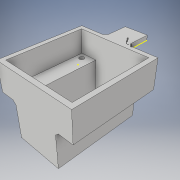
# Autodesk Inventor part: obudowa_baza
Saved by Autodesk Inventor 2019 (Build 230136000, 136)
## iProperties
Created: 2019-08-12
Part Number: obudowa_baza
Material: Ogólny
Document SubType Name: Modeling
Designer: mikol
Density: 1 g/cm^3
Appearance: Domyślna
Author: mikol
Autodesk Inventor part; units mm, degrees
ref_plane "YZ Plane" through (0, 0, 0) normal (1, 0, 0) x (0, 1, 0)
ref_plane "XZ Plane" through (0, 0, 0) normal (0, 1, 0) x (-1, 0, 0)
ref_plane "XY Plane" through (0, 0, 0) normal (0, 0, 1) x (1, 0, 0)
sketch "Sketch1" plane through (0, 0, 0) normal (0, 1, 0) x (-1, 0, 0)
  circle A0 centre (0, 12.75) radius 8.05
  circle A1 centre (0, -12.75) radius 8.05
  line L0 (14.5, 27) -> (-14.5, 27)
  line L1 (-14.5, 27) -> (-14.5, -27)
  line L2 (-14.5, -27) -> (14.5, -27)
  line L3 (14.5, -27) -> (14.5, 27)
  line L4 (14.5, 27) -> (-14.5, -27) construction
  line L5 (-14.5, 27) -> (14.5, -27) construction
  point P0 (0, 0)
  dimension "d0" = 16.1
  dimension "d1" = 16.1
  dimension "d2" = 25.5
  dimension "d3" = 29
  dimension "d4" = 54
  dimension "d5" = 14.5
  dimension "d6" = 14.5
  dimension "d7" = 14.25
  dimension "d8" = 14.25
  constraints: 12 end point, 2 centre point, 2 midpoint, 2 parallel, 1 horizontal, 1 perpendicular
  measures "d0" diameter of A0
  measures "d1" diameter of A1
  measures "d2" distance of A1.centre A0.centre
  measures "d3" distance of L2.end L1.end
  measures "d4" distance of L1.end L0.end
  measures "d5" distance from line of L3 A0.centre
  measures "d6" distance from line of A1.centre L3
  measures "d7" distance from line of L2 A1.centre
  measures "d8" distance from line of L0 A0.centre
extrude "Extrusion1" add sketch "Sketch1" along normal blind 3
sketch "Sketch2" plane through (0, 3, 0) normal (0, 1, 0) x (1, 0, 0)
  line L0 (-11.5, -24) -> (11.5, -24)
  line L1 (11.5, -24) -> (11.5, 24)
  line L2 (11.5, 24) -> (-11.5, 24)
  line L3 (-11.5, 24) -> (-11.5, -24)
  line L4 (-11.5, -24) -> (11.5, 24) construction
  line L5 (11.5, -24) -> (-11.5, 24) construction
  line L6 (14.5, -27) -> (14.5, 27) projected
  line L7 (-14.5, -27) -> (14.5, -27)
  line L8 (14.5, -27) -> (14.5, 27)
  line L9 (14.5, 27) -> (-14.5, 27)
  line L10 (-14.5, 27) -> (-14.5, -27)
  line L11 (-14.5, -27) -> (14.5, 27) construction
  line L12 (14.5, -27) -> (-14.5, 27) construction
  point P0 (0, 0)
  dimension "d11" = 23
  dimension "d12" = 48
  constraints: 24 end point, 4 midpoint, 4 parallel, 2 horizontal, 2 perpendicular
  measures "d11" distance of L2.end L1.end
  measures "d12" distance of L1.end L0.end
extrude "Extrusion2" add sketch "Sketch2" along normal blind 25
sketch "Sketch3" plane through (0, 28, 0) normal (0, 1, 0) x (1, 0, 0)
  line L0 (-25.5, 27) -> (25.5, 27)
  line L1 (25.5, 27) -> (25.5, -27)
  line L2 (25.5, -27) -> (-25.5, -27)
  line L3 (-25.5, -27) -> (-25.5, 27)
  line L4 (-25.5, 27) -> (25.5, -27) construction
  line L5 (25.5, 27) -> (-25.5, -27) construction
  line L6 (14.5, -27) -> (14.5, 27) projected
  line L7 (-14.5, 27) -> (14.5, 27)
  line L8 (14.5, 27) -> (14.5, -27)
  line L9 (14.5, -27) -> (-14.5, -27)
  line L10 (-14.5, -27) -> (-14.5, 27)
  line L11 (-14.5, 27) -> (14.5, -27) construction
  line L12 (14.5, 27) -> (-14.5, -27) construction
  point P0 (0, 0)
  dimension "d15" = 51
  constraints: 24 end point, 4 midpoint, 4 parallel, 2 horizontal, 2 perpendicular
  measures "d15" distance of L1.end L2.end
extrude "Extrusion3" add sketch "Sketch3" against normal blind 3 contours L0 L10 L2 L3 | L0 L1 L2 L6
sketch "Sketch4" plane through (0, 28, 0) normal (0, 1, 0) x (1, 0, 0)
  line L0 (-25.5, -27) -> (25.5, -27) projected
  line L1 (-25.5, 27) -> (25.5, 27)
  line L2 (25.5, 27) -> (25.5, -27)
  line L3 (25.5, -27) -> (-25.5, -27)
  line L4 (-25.5, -27) -> (-25.5, 27)
  line L5 (-25.5, 27) -> (25.5, -27) construction
  line L6 (25.5, 27) -> (-25.5, -27) construction
  line L7 (-22.5, 24) -> (22.5, 24)
  line L8 (22.5, 24) -> (22.5, -24)
  line L9 (22.5, -24) -> (-22.5, -24)
  line L10 (-22.5, -24) -> (-22.5, 24)
  line L11 (-22.5, 24) -> (22.5, -24) construction
  line L12 (22.5, 24) -> (-22.5, -24) construction
  point P0 (0, 0)
  dimension "d18" = 45
  dimension "d19" = 48
  constraints: 24 end point, 4 midpoint, 4 parallel, 2 horizontal, 2 perpendicular
  measures "d18" distance of L8.end L9.end
  measures "d19" distance of L7.end L8.end
extrude "Extrusion4" add sketch "Sketch4" along normal blind 15
sketch "Sketch5" plane through (0, 28, 0) normal (0, 1, 0) x (1, 0, 0)
  line L0 (-11.5, 24) -> (-22.5, 24) projected
  line L1 (-22.5, 24) -> (-22.5, -24) projected
  line L2 (-22.5, -24) -> (-11.5, -24) projected
  line L3 (-11.5, -24) -> (-11.5, 24) projected
  line L4 (22.5, 24) -> (11.5, 24) projected
  line L5 (11.5, 24) -> (11.5, -24) projected
  line L6 (11.5, -24) -> (22.5, -24) projected
  line L7 (22.5, -24) -> (22.5, 24) projected
  circle A0 centre (18.5, 20) radius 1.75
  line L8 (14.5, 27) -> (14.5, -27) projected
  line L9 (14.5, 27) -> (25.5, 27) projected
  line L10 (25.5, 27) -> (25.5, -27) projected
  line L11 (25.5, -27) -> (14.5, -27) projected
  line L12 (-11.5, 24) -> (-11.5, -24) projected
  line L13 (-11.5, -24) -> (11.5, -24) projected
  line L14 (11.5, -24) -> (11.5, 24) projected
  line L15 (11.5, 24) -> (-11.5, 24) projected
  circle A1 centre (0, 12.75) radius 8.05 projected
  circle A2 centre (0, -12.75) radius 8.05 projected
  circle A3 centre (18.5, -20) radius 1.75
  circle A4 centre (-18.5, 20) radius 1.75
  circle A5 centre (-18.5, -20) radius 1.75
  point P0 (0, 0)
  dimension "d22" = 3.5
  dimension "d23" = 4
  dimension "d24" = 4
  dimension "d25" = 4
  dimension "d28" = 40
  dimension "d31" = 37
  dimension "d53" = 4
  constraints: 4 centre point, 1 horizontal, 1 vertical, 6 other
  measures "d22" diameter of A0
  measures "d23" distance from line of L7 A0.centre
  measures "d24" distance from line of L8 A0.centre
  measures "d25" distance from line of L4 A0.centre
  measures "d28" distance of A0.centre A3.centre
  measures "d31" distance of A0.centre A4.centre
  measures "d53" distance from line of L6 A3.centre
extrude "Extrusion5" cut sketch "Sketch5" against normal blind 10 contours A0 | A3 | A4 | A5
chamfer "Chamfer1" distance 2 angle 45 4 edges at (-14.5, 0, 0) (14.5, 0, 0) (0, 0, 27) (0, 0, -27)
chamfer "Chamfer2" distance 2 angle 45 2 edges at (-14.5, 25, 0) (14.5, 25, 0)
sketch "Sketch6" plane through (0, 25, 0) normal (0, -1, 0) x (1, 0, 0)
  line L0 (-16.5, 27) -> (-16.5, -27) projected
  circle A0 centre (-18.5, -20) radius 1.75 projected
  circle A1 centre (-18.5, 20) radius 1.75 projected
  line L1 (-16.5, 27) -> (-25.5, 27) projected
  line L2 (-25.5, 27) -> (-25.5, -27) projected
  line L3 (-25.5, -27) -> (-16.5, -27) projected
  line L4 (16.5, -27) -> (16.5, 27) projected
  circle A2 centre (18.5, -20) radius 1.75 projected
  line L5 (16.5, -27) -> (25.5, -27) projected
  line L6 (25.5, -27) -> (25.5, 27) projected
  line L7 (25.5, 27) -> (16.5, 27) projected
  circle A3 centre (18.5, 20) radius 1.75 projected
  circle A4 centre (18.5, -20) radius 3
  circle A5 centre (18.5, 20) radius 3
  circle A6 centre (-18.5, -20) radius 3
  circle A7 centre (-18.5, 20) radius 3
  point P0 (0, 0)
  dimension "d42" = 6
  dimension "d45" = 40
  dimension "d48" = 37
  constraints: 4 centre point, 1 coincident, 1 horizontal, 1 vertical, 6 other
  measures "d42" diameter of A4
  measures "d45" distance of A4.centre A5.centre
  measures "d48" distance of A4.centre A6.centre
extrude "Extrusion6" cut sketch "Sketch6" along normal blind 10 contours A7 L0 | L0 A7 | A6 L0 | L0 A6 | A0 | A1 | A4 L4 | L4 A4 | A5 L4 | L4 A5 | A2 | A3
sketch "Sketch7" plane through (25.5, 43, -27) normal (0, 0, -1) x (-1, 0, 0)
  line L0 (40, -41) -> (11, -41) projected
  line L1 (40, -41) -> (40, -20) projected
  line L2 (42, -18) -> (40, -20) projected
  line L3 (51, -18) -> (42, -18) projected
  line L4 (51, 0) -> (51, -18) projected
  line L5 (0, 0) -> (51, 0) projected
  line L6 (0, -18) -> (0, 0) projected
  line L7 (9, -18) -> (0, -18) projected
  line L8 (11, -20) -> (9, -18) projected
  line L9 (11, -41) -> (11, -20) projected
  line L10 (0, 0) -> (51, 0) projected
  line L11 (18, 0) -> (33, 0)
  line L12 (33, 0) -> (33, -3)
  line L13 (33, -3) -> (18, -3)
  line L14 (18, -3) -> (18, 0)
  point P0 (25.5, -43)
  dimension "d54" = 15
  dimension "d55" = 3
  dimension "d56" = 18
  dimension "d57" = 18
  constraints: 8 end point, 2 parallel, 1 horizontal, 1 perpendicular, 1 point on line
  measures "d54" distance of L12.end L13.end
  measures "d55" distance of L11.end L12.end
  measures "d56" distance between parallel lines of L4 L12
  measures "d57" distance between parallel lines of L6 L14
extrude "Extrusion7" add sketch "Sketch7" along normal blind 16 contours L12 L13 L14 L5
chamfer "Chamfer3" distance 2 angle 45 3 edges at (0, 40, -27) (-7.5, 41.5, -27) (7.5, 41.5, -27)
sketch "Sketch8" plane through (-7.5, 40, -43) normal (0, -1, 0) x (1, 0, 0)
  line L0 (0, 14) -> (15, 14) projected
  line L1 (0, 14) -> (0, 0) projected
  line L2 (15, 0) -> (0, 0) projected
  line L3 (15, 14) -> (15, 0) projected
  circle A0 centre (7.5, 7) radius 3
  point P0 (7.5, 43)
  dimension "d63" = 6
  constraints: 1 centre point
  measures "d63" diameter of A0
equation "\"d7\" = d8"
equation "\"d23\" = d24"
equation "\"d25\" = d53"
equation "\"d56\" = d57"
body "Solid1"
